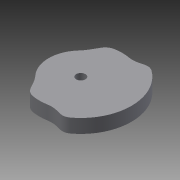
# Autodesk Inventor part: 重要
Saved by Autodesk Inventor 2013 (Build 170138000, 138)
## iProperties
Created: 2012-09-25
Part Number: 重要
Material: 常规
Document SubType Name: Modeling
Designer: Zhensheng
Density: 1 g/cm^3
Mass: 0.957115 g
Surface Area: 11.492 cm^2
Volume: 0.957115 cm^3
Author: Zhensheng
Autodesk Inventor part; units mm, degrees
ref_plane "YZ Plane" through (0, 0, 0) normal (1, 0, 0) x (0, 1, 0)
ref_plane "XZ Plane" through (0, 0, 0) normal (0, 1, 0) x (-1, 0, 0)
ref_plane "XY Plane" through (0, 0, 0) normal (0, 0, 1) x (1, 0, 0)
sketch "草图1" plane through (0, 0, 0) normal (0, 0, 1) x (1, 0, 0)
  line L0 (0, 0) -> (0, 45) construction
  arc A0 (7.7977, 44.3192) -> (0, 45) centre (0, 0) ccw
  line L1 (0, 0) -> (13.1567, 43.0337) construction
  line L2 (0, 0) -> (0, 45) construction
  arc A1 (32.563, -44.3244) -> (32.563, 44.3244) centre (0, 0) ccw
  line L3 (0, 0) -> (16.0804, -52.5968) construction
  line L4 (0, 0) -> (16.0804, 52.5968) construction
  arc A2 (0, -45) -> (7.7977, -44.3192) centre (0, 0) ccw
  arc A3 (0, 45) -> (-7.7977, 44.3192) centre (0, 0) ccw
  arc A4 (-7.7977, -44.3192) -> (0, -45) centre (0, 0) ccw
  line L5 (0, 0) -> (45, 0) construction
  arc A5 (7.7977, 44.3192) -> (18.5563, 44.729) centre (12.2262, 69.489) ccw
  arc A6 (32.563, 44.3244) -> (23.7003, 46.0441) centre (26.3144, 35.8188) ccw
  line L6 (18.5563, 44.729) -> (23.7003, 46.0441)
  arc A7 (18.5563, -44.729) -> (7.7977, -44.3192) centre (12.2262, -69.489) ccw
  arc A8 (23.7003, -46.0441) -> (32.563, -44.3244) centre (26.3144, -35.8188) ccw
  line L7 (18.5563, -44.729) -> (23.7003, -46.0441)
  line L8 (0, 0) -> (-13.1567, 43.0337) construction
  line L9 (0, 0) -> (-13.1567, -43.0337) construction
  arc A9 (-25.925, 23.5137) -> (-25.925, -23.5137) centre (0, 0) ccw
  arc A10 (-7.7977, 44.3192) -> (-16.3105, 38.3374) centre (-5.674, 32.2489) ccw
  arc A11 (-25.925, 23.5137) -> (-20.6001, 30.8435) centre (-56.9437, 51.6471) ccw
  line L10 (-16.3105, 38.3374) -> (-20.6001, 30.8435)
  arc A12 (-16.3105, -38.3374) -> (-7.7977, -44.3192) centre (-5.674, -32.2489) ccw
  arc A13 (-20.6001, -30.8435) -> (-25.925, -23.5137) centre (-56.9437, -51.6471) ccw
  line L11 (-16.3105, -38.3374) -> (-20.6001, -30.8435)
  arc A14 (-7.7977, -44.3192) -> (7.7977, -44.3192) centre (0, 0) ccw construction
  arc A15 (13.1567, -43.0337) -> (-13.1567, -43.0337) centre (0, 0) ccw construction
  circle A16 centre (0, 0) radius 5
  dimension "d43" = 17
  dimension "d45" = 55
  dimension "d46" = 146
  dimension "d49" = 25.5563
  dimension "d50" = 5.3094
  dimension "d51" = 10.5541
  dimension "d52" = 17
  dimension "d53" = 34
  dimension "d54" = 35
  dimension "d55" = 12.2558
  dimension "d56" = 8.6348
  dimension "d57" = 41.8766
  dimension "凸轮孔直径" = 10
  constraints: 35 point on circle, 24 end point, 17 centre point, 14 symmetric about line, 7 coincident, 7 tangent, 1 collinear, 1 point on line, 1 vertical, 7 other
  measures "d43" angle of L1 L2
  measures "d45" radius of A1
  measures "d46" angle of L3 L4
  measures "d49" radius of A5
  measures "d50" distance of L6.start L6.end
  measures "d51" radius of A6
  measures "d52" angle of L8 L0
  measures "d53" angle of L9 L3
  measures "d54" radius of A9
  measures "d55" radius of A10
  measures "d56" distance of L10.start L10.end
  measures "d57" radius of A11
  measures "凸轮孔直径" diameter of A16
extrude "拉伸3" add sketch "草图1" along normal mid plane 15
